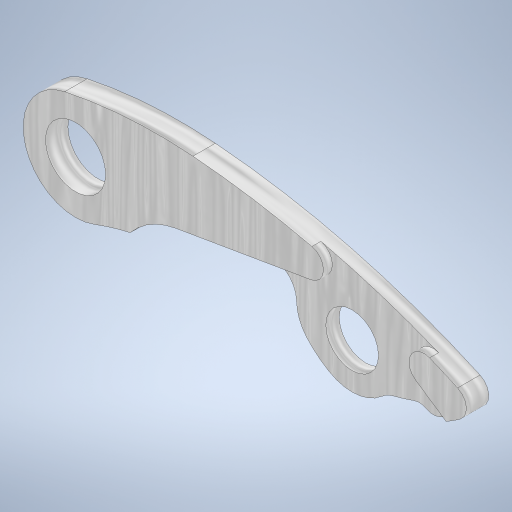
# Autodesk Inventor part: 揺動節
Saved by Autodesk Inventor 2023 (Build 270158030, 158C)
## iProperties
Created: 2022-01-09
Part Number: 揺動節
Material: アルミニウム 7075
Document SubType Name: Modeling
Designer: acps
Density: 2.81 g/cm^3
Appearance: サテン - ブラシ仕上げ 重厚
Mass: 3.82465 g
Surface Area: 15.3772 cm^2
Volume: 1.36109 cm^3
Author: acps
Autodesk Inventor part; units mm, degrees
ref_plane "YZ Plane" through (0, 0, 0) normal (1, 0, 0) x (0, 1, 0)
ref_plane "XZ Plane" through (0, 0, 0) normal (0, 1, 0) x (-1, 0, 0)
ref_plane "XY Plane" through (0, 0, 0) normal (0, 0, 1) x (1, 0, 0)
sketch "Sketch1" plane through (0, 0, 0) normal (0, 0, 1) x (1, 0, 0)
  line L0 (65.359, 13) -> (101.145, 9.0808) construction
  circle A0 centre (65.359, 13) radius 3 construction
  circle A1 centre (65.359, 13) radius 4.025
  circle A2 centre (65.359, 13) radius 7
  arc A3 (103.9065, 14.4076) -> (101.5853, 15.5481) centre (76.292, -38.8601) ccw construction
  arc A4 (98.0987, 3.9117) -> (67.8539, 6.4597) centre (80.3286, -26.2417) ccw
  circle A5 centre (101.145, 9.0808) radius 2.5 construction
  circle A6 centre (101.145, 9.0808) radius 3.525
  circle A7 centre (101.145, 9.0808) radius 6
  line L1 (101.145, 9.0808) -> (116.8532, -6.3223) construction
  circle A8 centre (116.8532, -6.3223) radius 10 construction
  circle A9 centre (116.8532, -6.3223) radius 7.025 construction
  line L2 (104.4969, 14.0572) -> (122.4397, 1.9718) construction
  line L3 (96.2353, 5.6319) -> (108.6703, -12.0703) construction
  line L4 (121.8748, 2.4728) -> (123.0794, 1.6615) construction
  arc A10 (101.4998, 3.0913) -> (116.7565, 8.3414) centre (99.726, 33.0388) ccw
  arc A11 (116.4477, 11.8091) -> (81.0555, 20.9505) centre (72.64, -84.7149) ccw
  arc A12 (116.7565, 8.3414) -> (116.4477, 11.8091) centre (115.6212, 9.9879) ccw
  line L5 (65.359, 13) -> (100, 0) construction
  arc A13 (112.7035, 13.4223) -> (110.8303, 9.9119) centre (111.9476, 11.5707) ccw
  line L6 (101.145, 9.0808) -> (80.4889, 1.5095) construction
  circle A14 centre (80.4889, 1.5095) radius 7.025 construction
  circle A15 centre (80.4889, 1.5095) radius 10 construction
  line L7 (110.8303, 9.9119) -> (114.9091, 7.1646)
  arc A16 (81.0555, 20.9505) -> (63.915, 19.8494) centre (76.292, -38.8601) ccw
  arc A17 (101.5853, 15.5481) -> (81.0555, 20.9505) centre (76.292, -38.8601) ccw construction
  line L8 (78.8119, 11.3678) -> (100.1388, 14.9958) construction
  line L9 (78.7951, 11.4664) -> (105.6086, 16.0277)
  arc A18 (78.7951, 11.4664) -> (72.6773, 7.9118) centre (80.4889, 1.5095) ccw
  circle A19 centre (108.9991, 1.3793) radius 2.85 construction
  arc A20 (98.9782, 4.5486) -> (109.436, 6.244) centre (99.726, 33.0388) ccw
  arc A21 (111.0687, 6.1229) -> (109.436, 6.244) centre (110.1175, 4.3636) ccw
  line L10 (111.3917, 5.9167) -> (113.93, 4.207) construction
  arc A22 (93.7202, 9.8939) -> (89.6334, 13.3102) centre (90.2203, 9.8597) ccw
  arc A23 (111.0687, 6.1229) -> (112.8982, 6.0853) centre (112.02, 7.8822) ccw
  arc A24 (96.8456, 14.537) -> (96.9692, 18.4553) centre (96.5101, 16.5087) ccw
  arc A25 (93.7202, 9.8939) -> (98.9782, 4.5486) centre (99.1199, 9.9468) ccw
  arc A26 (106.7234, 5.4112) -> (105.0813, 4.5525) centre (107.7055, 1.5336) ccw
  arc A27 (95.0804, 6.3632) -> (98.2329, 3.8349) centre (104.0571, 14.3267) ccw
  point P0 (0, 0)
  point P1 (104.5045, 16.3824)
  point P2 (75.0442, 8.3571)
  point P3 (105.6964, 5.1712)
  point P4 (95.4674, 18.798)
  point P5 (96.589, 5.1766)
  point P6 (97.8471, 4.0585)
  dimension "d10" = 12
  dimension "d57" = 20
  dimension "d1" = 8.05
  dimension "d2" = 6
  dimension "d3" = 14
  dimension "d4" = 60
  dimension "d5" = 35
  dimension "d8" = 22
  dimension "d11" = 7.05
  dimension "d12" = 20
  dimension "d13" = 14.05
  dimension "d15" = 0.1
  dimension "d16" = 30
  dimension "d17" = 5
  dimension "d18" = 2
  dimension "d19" = 106
  dimension "d21" = 121
  dimension "d46" = 13
  dimension "d47" = 37
  dimension "d48" = 18
  dimension "d50" = 0
  dimension "d51" = 100
  dimension "d53" = 2
  dimension "d54" = 4
  dimension "d55" = 22
  dimension "d56" = 14.05
  dimension "d65" = 14.32
  dimension "d68" = 26.38
  dimension "d69" = 0.1
  dimension "d70" = 0.1
  dimension "d72" = 36
  dimension "d77" = 5.7
  dimension "d78" = 2
  dimension "d79" = 3
  dimension "d86" = 1.5
  dimension "d87" = 2
  dimension "d88" = 2
  dimension "d90" = 5.4
  dimension "d91" = 3.5
  dimension "d92" = 4
  dimension "d93" = 12
  constraints: 49 point on circle, 26 centre point, 22 end point, 19 tangent, 10 coincident, 5 point on line, 3 parallel, 1 concentric, 1 equal radius, 1 midpoint, 23 other
  measures "d1" diameter of A1
  measures "d2" diameter of A0
  measures "d3" diameter of A2
  measures "d4" radius of A3
  measures "d5" radius of A4
  measures "d8" distance of L1.start L1.end
  measures "d11" diameter of A6
  measures "d12" diameter of A8
  measures "d13" diameter of A9
  measures "d15" distance between parallel lines of L2 L4
  measures "d16" radius of A10
  measures "d17" diameter of A5
  measures "d18" radius of A12
  measures "d19" radius of A11
  measures "d46" vertical distance of point (0, 0) L0.start
  measures "d47" distance of L5.start L5.end
  measures "d48" distance of L5.end A9.centre
  measures "d50" vertical distance of point (0, 0) L5.end
  measures "d51" distance of point (0, 0) L5.end
  measures "d53" radius of A13
  measures "d54" distance of A12.centre A13.centre
  measures "d55" distance of L1.start L6.end
  measures "d56" diameter of A14
  measures "d65" angle of L5 L0
  measures "d68" angle of L6 L0
  measures "d69" distance between parallel lines of L8 L9
  measures "d72" distance of L0.end L0.start
  measures "d77" diameter of A19
  measures "d78" radius of A21
  measures "d79" distance between parallel lines of L10 L7
  measures "d86" radial gap between concentric circles of A10 A20
  measures "d87" radius of A23
  measures "d88" radius of A24
  measures "d90" radius of A25
  measures "d91" radius of A22
  measures "d92" radius of A26
  measures "d93" radius of A27
extrude "Extrusion7" add sketch "Sketch1" along normal blind 3 contours A2 | A2 A16 A11 A24 L9 A18 A4 | A11 A12 A10 L7 A13
extrude "Extrusion8" add sketch "Sketch1" along normal blind 1.8 contours A11 L9 A24 | A7 A25 A20 | A27 A25 A7 | A11 A13 L7 A10 A23 A21 A20 A7 A25 A22 L9 | A7 A20 A25 | A7 A20 A26
sketch "Sketch4" plane through (0, 0, 3) normal (0, 0, 1) x (1, 0, 0)
  arc A0 (96.8456, 14.537) -> (96.9692, 18.4553) centre (96.5101, 16.5087) ccw projected
  circle A1 centre (65.359, 13) radius 4.025 projected
  arc A2 (112.7035, 13.4223) -> (96.9692, 18.4553) centre (72.64, -84.7149) ccw construction
  arc A3 (96.8456, 14.537) -> (96.9692, 18.4553) centre (96.5101, 16.5087) ccw projected
  line L0 (89.6334, 13.3102) -> (96.8456, 14.537) projected
  arc A4 (93.7202, 9.8939) -> (89.6334, 13.3102) centre (90.2203, 9.8597) ccw construction
  arc A5 (93.7202, 9.8939) -> (95.0804, 6.3632) centre (99.1199, 9.9468) ccw construction
  arc A6 (95.0804, 6.3632) -> (97.8471, 4.0585) centre (104.0571, 14.3267) ccw construction
  arc A7 (98.0987, 3.9117) -> (97.8471, 4.0585) centre (80.3286, -26.2417) ccw construction
  arc A8 (98.0987, 3.9117) -> (105.0813, 4.5525) centre (101.145, 9.0808) ccw construction
  arc A9 (106.7234, 5.4112) -> (105.0813, 4.5525) centre (107.7055, 1.5336) ccw construction
  arc A10 (106.7234, 5.4112) -> (109.436, 6.244) centre (99.726, 33.0388) ccw construction
  arc A11 (111.0687, 6.1229) -> (109.436, 6.244) centre (110.1175, 4.3636) ccw construction
  arc A12 (111.0687, 6.1229) -> (112.8982, 6.0853) centre (112.02, 7.8822) ccw construction
  arc A13 (112.8982, 6.0853) -> (114.9091, 7.1646) centre (99.726, 33.0388) ccw construction
  line L1 (110.8303, 9.9119) -> (114.9091, 7.1646) projected
  arc A14 (112.7035, 13.4223) -> (110.8303, 9.9119) centre (111.9476, 11.5707) ccw projected
  circle A15 centre (101.145, 9.0808) radius 3.525 projected
  arc A16 (112.7035, 13.4223) -> (110.8303, 9.9119) centre (111.9476, 11.5707) ccw projected
  line L2 (110.8303, 9.9119) -> (114.9091, 7.1646) projected
  line L3 (110.8303, 9.9119) -> (114.9091, 7.1646) projected
  arc A17 (89.6334, 13.3102) -> (88.9291, 11.8348) centre (89.8011, 12.3243) ccw
  arc A18 (88.9291, 11.8348) -> (114.8991, 5.4992) centre (104.8698, 20.7826) ccw
  arc A19 (114.8991, 5.4992) -> (114.9091, 7.1646) centre (114.3504, 6.3352) ccw
  arc A20 (112.7035, 13.4223) -> (96.9692, 18.4553) centre (72.64, -84.7149) ccw projected
  arc A21 (97.5034, 20.3811) -> (96.9692, 18.4553) centre (97.1987, 19.4286) ccw
  arc A22 (112.7035, 13.4223) -> (113.3862, 15.3006) centre (113.0815, 14.3482) ccw
  line L4 (97.5034, 20.3811) -> (113.3862, 15.3006)
  arc A23 (112.7035, 13.4223) -> (110.8303, 9.9119) centre (111.9476, 11.5707) ccw projected
  arc A24 (96.8456, 14.537) -> (96.9692, 18.4553) centre (96.5101, 16.5087) ccw projected
  arc A25 (93.7202, 9.8939) -> (89.6334, 13.3102) centre (90.2203, 9.8597) ccw projected
  line L5 (89.6334, 13.3102) -> (96.8456, 14.537)
  line L6 (89.6334, 13.3102) -> (96.8456, 14.537)
  circle A26 centre (65.359, 13) radius 4.025 projected
  circle A27 centre (101.145, 9.0808) radius 3.525 projected
  arc A28 (116.4477, 11.8091) -> (81.0555, 20.9505) centre (72.64, -84.7149) ccw projected
  arc A29 (116.7565, 8.3414) -> (116.4477, 11.8091) centre (115.6212, 9.9879) ccw projected
  arc A30 (112.8982, 6.0853) -> (116.7565, 8.3414) centre (99.726, 33.0388) ccw projected
  arc A31 (111.0687, 6.1229) -> (112.8982, 6.0853) centre (112.02, 7.8822) ccw projected
  arc A32 (111.0687, 6.1229) -> (109.436, 6.244) centre (110.1175, 4.3636) ccw projected
  arc A33 (106.7234, 5.4112) -> (109.436, 6.244) centre (99.726, 33.0388) ccw projected
  arc A34 (106.7234, 5.4112) -> (105.0813, 4.5525) centre (107.7055, 1.5336) ccw projected
  arc A35 (98.0987, 3.9117) -> (105.0813, 4.5525) centre (101.145, 9.0808) ccw projected
  arc A36 (98.0987, 3.9117) -> (97.8471, 4.0585) centre (80.3286, -26.2417) ccw projected
  arc A37 (95.0804, 6.3632) -> (97.8471, 4.0585) centre (104.0571, 14.3267) ccw projected
  arc A38 (93.7202, 9.8939) -> (95.0804, 6.3632) centre (99.1199, 9.9468) ccw projected
  arc A39 (93.7202, 9.8939) -> (89.6334, 13.3102) centre (90.2203, 9.8597) ccw projected
  line L7 (78.7951, 11.4664) -> (89.6334, 13.3102) projected
  arc A40 (78.7951, 11.4664) -> (72.6773, 7.9118) centre (80.4889, 1.5095) ccw projected
  arc A41 (72.6773, 7.9118) -> (67.8539, 6.4597) centre (80.3286, -26.2417) ccw projected
  arc A42 (63.915, 19.8494) -> (67.8539, 6.4597) centre (65.359, 13) ccw projected
  arc A43 (81.0555, 20.9505) -> (63.915, 19.8494) centre (76.292, -38.8601) ccw projected
  point P0 (0, 0)
  dimension "d94" = 1
  dimension "d95" = 1
  dimension "d96" = 1
  dimension "d97" = 1
  constraints: 11 point on circle, 9 tangent, 8 centre point, 6 end point
  measures "d94" radius of A17
  measures "d95" radius of A19
  measures "d96" radius of A21
  measures "d97" radius of A22
body "Solid4"
